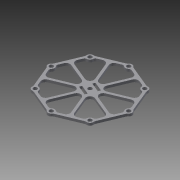
# Autodesk Inventor part: RPiConnector
Saved by Autodesk Inventor 2014 SP1 (Build 180222100, 222)
## iProperties
Created: 2014-07-30
Part Number: RPiConnector
Material: Generic
Document SubType Name: Modeling
Designer: Ryan
Density: 1 g/cm^3
Appearance: Default
Author: Ryan
Autodesk Inventor part; units mm, degrees
ref_plane "YZ Plane" through (0, 0, 0) normal (1, 0, 0) x (0, 1, 0)
ref_plane "XZ Plane" through (0, 0, 0) normal (0, 1, 0) x (-1, 0, 0)
ref_plane "XY Plane" through (0, 0, 0) normal (0, 0, 1) x (1, 0, 0)
sketch "Middle Plate" plane through (0, 0, 0) normal (0, 0, 1) x (1, 0, 0)
  circle A0 centre (54.1802, 86) radius 1.6
  circle A1 centre (63.5, 108.5) radius 1.6
  circle A2 centre (86, 117.8198) radius 1.6
  circle A3 centre (108.5, 108.5) radius 1.6
  circle A4 centre (117.8198, 86) radius 1.6
  circle A5 centre (108.5, 63.5) radius 1.6
  circle A6 centre (63.5, 63.5) radius 1.6
  circle A7 centre (86, 54.1802) radius 1.6
  arc A8 (56.1767, 84.1823) -> (56.1767, 87.8177) centre (54.1802, 86) ccw
  arc A9 (55.8078, 89.9295) -> (56.1767, 87.8177) centre (57.6556, 89.1641) ccw
  arc A10 (56.1767, 84.1823) -> (55.8078, 82.0705) centre (57.6556, 82.8359) ccw
  arc A11 (63.6264, 105.803) -> (66.197, 108.3735) centre (63.5, 108.5) ccw
  arc A12 (63.6264, 105.803) -> (61.8724, 104.5705) centre (63.7201, 103.8052) ccw
  arc A13 (67.4295, 110.1276) -> (66.197, 108.3735) centre (68.1948, 108.2799) ccw
  arc A14 (84.1823, 115.8233) -> (87.8177, 115.8233) centre (86, 117.8198) ccw
  arc A15 (89.9295, 116.1922) -> (87.8177, 115.8233) centre (89.1641, 114.3444) ccw
  arc A16 (84.1823, 115.8233) -> (82.0705, 116.1922) centre (82.8359, 114.3444) ccw
  arc A17 (105.803, 108.3735) -> (108.3735, 105.803) centre (108.5, 108.5) ccw
  arc A18 (110.1276, 104.5705) -> (108.3735, 105.803) centre (108.2799, 103.8052) ccw
  arc A19 (105.803, 108.3735) -> (104.5705, 110.1276) centre (103.8052, 108.2799) ccw
  arc A20 (115.8233, 87.8177) -> (115.8233, 84.1823) centre (117.8198, 86) ccw
  arc A21 (116.1922, 82.0705) -> (115.8233, 84.1823) centre (114.3444, 82.8359) ccw
  arc A22 (115.8233, 87.8177) -> (116.1922, 89.9295) centre (114.3444, 89.1641) ccw
  arc A23 (66.197, 63.6265) -> (63.6264, 66.197) centre (63.5, 63.5) ccw
  arc A24 (61.8724, 67.4295) -> (63.6264, 66.197) centre (63.7201, 68.1948) ccw
  arc A25 (66.197, 63.6265) -> (67.4295, 61.8724) centre (68.1948, 63.7201) ccw
  arc A26 (87.8177, 56.1767) -> (84.1823, 56.1767) centre (86, 54.1802) ccw
  arc A27 (82.0705, 55.8078) -> (84.1823, 56.1767) centre (82.8359, 57.6556) ccw
  arc A28 (87.8177, 56.1767) -> (89.9295, 55.8078) centre (89.1641, 57.6556) ccw
  arc A29 (108.3735, 66.197) -> (105.803, 63.6265) centre (108.5, 63.5) ccw
  arc A30 (104.5705, 61.8724) -> (105.803, 63.6265) centre (103.8052, 63.7201) ccw
  arc A31 (108.3735, 66.197) -> (110.1276, 67.4295) centre (108.2799, 68.1948) ccw
  line L0 (55.8078, 82.0705) -> (61.8724, 67.4295)
  line L1 (67.4295, 61.8724) -> (82.0705, 55.8078)
  line L2 (89.9295, 55.8078) -> (104.5705, 61.8724)
  line L3 (110.1276, 67.4295) -> (116.1922, 82.0705)
  line L4 (116.1922, 89.9295) -> (110.1276, 104.5705)
  line L5 (104.5705, 110.1276) -> (89.9295, 116.1922)
  line L6 (82.0705, 116.1922) -> (67.4295, 110.1276)
  line L7 (61.8724, 104.5705) -> (55.8078, 89.9295)
  point P0 (86, 86)
sketch "Sketch1" plane through (0, 0, 0) normal (0, 1, 0) x (-1, 0, 0)
  arc A0 (66.197, 63.6265) -> (67.4295, 61.8724) centre (68.1948, 63.7201) ccw
  arc A1 (61.8724, 67.4295) -> (63.6264, 66.197) centre (63.7201, 68.1948) ccw
  line L0 (61.8724, 67.4295) -> (60.0246, 66.6641)
  line L1 (67.4295, 61.8724) -> (66.6641, 60.0246)
  arc A2 (82.0705, 55.8078) -> (84.1823, 56.1767) centre (82.8359, 57.6556) ccw
  arc A3 (87.8177, 56.1767) -> (89.9295, 55.8078) centre (89.1641, 57.6556) ccw
  arc A4 (104.5705, 61.8724) -> (105.803, 63.6265) centre (103.8052, 63.7201) ccw
  arc A5 (108.3735, 66.197) -> (110.1276, 67.4295) centre (108.2799, 68.1948) ccw
  line L2 (67.4295, 61.8724) -> (82.0705, 55.8078)
  line L3 (82.0705, 55.8078) -> (81.3052, 53.9601)
  line L4 (81.3052, 53.9601) -> (66.6641, 60.0246)
  line L5 (89.9295, 55.8078) -> (104.5705, 61.8724)
  arc A6 (56.1767, 84.1823) -> (55.8078, 82.0705) centre (57.6556, 82.8359) ccw
  arc A7 (55.8078, 89.9295) -> (56.1767, 87.8177) centre (57.6556, 89.1641) ccw
  arc A8 (63.6264, 105.803) -> (61.8724, 104.5705) centre (63.7201, 103.8052) ccw
  arc A9 (67.4295, 110.1276) -> (66.197, 108.3735) centre (68.1948, 108.2799) ccw
  arc A10 (84.1823, 115.8233) -> (82.0705, 116.1922) centre (82.8359, 114.3444) ccw
  arc A11 (89.9295, 116.1922) -> (87.8177, 115.8233) centre (89.1641, 114.3444) ccw
  arc A12 (105.803, 108.3735) -> (104.5705, 110.1276) centre (103.8052, 108.2799) ccw
  arc A13 (110.1276, 104.5705) -> (108.3735, 105.803) centre (108.2799, 103.8052) ccw
  arc A14 (115.8233, 87.8177) -> (116.1922, 89.9295) centre (114.3444, 89.1641) ccw
  arc A15 (116.1922, 82.0705) -> (115.8233, 84.1823) centre (114.3444, 82.8359) ccw
  line L6 (110.1276, 67.4295) -> (116.1922, 82.0705)
  line L7 (116.1922, 89.9295) -> (110.1276, 104.5705)
  line L8 (104.5705, 110.1276) -> (89.9295, 116.1922)
  line L9 (82.0705, 116.1922) -> (67.4295, 110.1276)
  line L10 (61.8724, 104.5705) -> (55.8078, 89.9295)
  line L11 (55.8078, 82.0705) -> (61.8724, 67.4295)
  line L12 (55.8078, 82.0705) -> (53.9601, 81.3052)
  line L13 (55.8078, 89.9295) -> (53.9601, 90.6948)
  line L14 (61.8724, 104.5705) -> (60.0246, 105.3359)
  line L15 (60.0246, 105.3359) -> (53.9601, 90.6948)
  line L16 (60.0246, 66.6641) -> (53.9601, 81.3052)
  line L17 (89.9295, 55.8078) -> (90.6948, 53.9601)
  line L18 (104.5705, 61.8724) -> (105.3359, 60.0246)
  line L19 (90.6948, 53.9601) -> (105.3359, 60.0246)
  line L20 (110.1276, 67.4295) -> (111.9754, 66.6641)
  line L21 (116.1922, 82.0705) -> (118.0399, 81.3052)
  line L22 (118.0399, 81.3052) -> (111.9754, 66.6641)
  line L23 (116.1922, 89.9295) -> (118.0399, 90.6948)
  line L24 (110.1276, 104.5705) -> (111.9754, 105.3359)
  line L25 (111.9754, 105.3359) -> (118.0399, 90.6948)
  line L26 (104.5705, 110.1276) -> (105.3359, 111.9754)
  line L27 (89.9295, 116.1922) -> (90.6948, 118.0399)
  line L28 (90.6948, 118.0399) -> (105.3359, 111.9754)
  line L29 (82.0705, 116.1922) -> (81.3052, 118.0399)
  line L30 (67.4295, 110.1276) -> (66.6641, 111.9754)
  line L31 (66.6641, 111.9754) -> (81.3052, 118.0399)
  line L32 (60.0246, 105.3359) -> (60.9581, 107.5896)
  line L33 (66.6641, 111.9754) -> (64.4104, 111.0419)
  line L34 (90.6948, 118.0399) -> (88.4411, 118.9734)
  line L35 (81.3052, 118.0399) -> (83.5589, 118.9734)
  line L36 (105.3359, 111.9754) -> (107.5896, 111.0419)
  line L37 (111.9754, 105.3359) -> (111.0419, 107.5896)
  line L38 (118.0399, 90.6948) -> (118.9734, 88.4411)
  line L39 (118.0399, 81.3052) -> (118.9734, 83.5589)
  line L40 (111.9754, 66.6641) -> (111.0419, 64.4104)
  line L41 (105.3359, 60.0246) -> (107.5896, 60.9581)
  line L42 (81.3052, 53.9601) -> (83.5589, 53.0266)
  line L43 (90.6948, 53.9601) -> (88.4411, 53.0266)
  line L44 (66.6641, 60.0246) -> (64.4104, 60.9581)
  line L45 (60.0246, 66.6641) -> (60.9581, 64.4104)
  line L46 (53.9601, 81.3052) -> (53.0266, 83.5589)
  line L47 (53.9601, 90.6948) -> (53.0266, 88.4411)
  circle A16 centre (54.1802, 86) radius 1.6
  circle A17 centre (63.5, 108.5) radius 1.6
  circle A18 centre (86, 117.8198) radius 1.6
  circle A19 centre (108.5, 108.5) radius 1.6
  circle A20 centre (117.8198, 86) radius 1.6
  circle A21 centre (108.5, 63.5) radius 1.6
  circle A22 centre (86, 54.1802) radius 1.6
  arc A23 (56.1767, 84.1823) -> (55.8078, 82.0705) centre (57.6556, 82.8359) ccw
  arc A24 (55.8078, 89.9295) -> (56.1767, 87.8177) centre (57.6556, 89.1641) ccw
  arc A25 (63.6264, 105.803) -> (61.8724, 104.5705) centre (63.7201, 103.8052) ccw
  arc A26 (67.4295, 110.1276) -> (66.197, 108.3735) centre (68.1948, 108.2799) ccw
  arc A27 (84.1823, 115.8233) -> (82.0705, 116.1922) centre (82.8359, 114.3444) ccw
  arc A28 (89.9295, 116.1922) -> (87.8177, 115.8233) centre (89.1641, 114.3444) ccw
  arc A29 (105.803, 108.3735) -> (104.5705, 110.1276) centre (103.8052, 108.2799) ccw
  arc A30 (110.1276, 104.5705) -> (108.3735, 105.803) centre (108.2799, 103.8052) ccw
  arc A31 (115.8233, 87.8177) -> (116.1922, 89.9295) centre (114.3444, 89.1641) ccw
  arc A32 (116.1922, 82.0705) -> (115.8233, 84.1823) centre (114.3444, 82.8359) ccw
  arc A33 (108.3735, 66.197) -> (110.1276, 67.4295) centre (108.2799, 68.1948) ccw
  arc A34 (104.5705, 61.8724) -> (105.803, 63.6265) centre (103.8052, 63.7201) ccw
  arc A35 (87.8177, 56.1767) -> (89.9295, 55.8078) centre (89.1641, 57.6556) ccw
  arc A36 (82.0705, 55.8078) -> (84.1823, 56.1767) centre (82.8359, 57.6556) ccw
  arc A37 (66.1912, 63.7184) -> (67.4295, 61.8724) centre (68.2018, 63.7288) ccw
  arc A38 (61.8724, 67.4295) -> (63.6264, 66.197) centre (63.7201, 68.1948) ccw
  arc A39 (87.8177, 56.1767) -> (84.1823, 56.1767) centre (86, 54.1802) ccw
  arc A40 (83.5589, 53.0266) -> (88.4411, 53.0266) centre (86, 54.1802) ccw
  arc A41 (66.1912, 63.7184) -> (63.6264, 66.197) centre (63.5, 63.5) ccw
  arc A42 (60.9581, 64.4104) -> (64.4104, 60.9581) centre (63.5, 63.5) ccw
  arc A43 (108.3735, 66.197) -> (105.803, 63.6265) centre (108.5, 63.5) ccw
  arc A44 (107.5896, 60.9581) -> (111.0419, 64.4104) centre (108.5, 63.5) ccw
  arc A45 (115.8233, 87.8177) -> (115.8233, 84.1823) centre (117.8198, 86) ccw
  arc A46 (118.9734, 83.5589) -> (118.9734, 88.4411) centre (117.8198, 86) ccw
  arc A47 (105.803, 108.3735) -> (108.3735, 105.803) centre (108.5, 108.5) ccw
  arc A48 (111.0419, 107.5896) -> (107.5896, 111.0419) centre (108.5, 108.5) ccw
  arc A49 (84.1823, 115.8233) -> (87.8177, 115.8233) centre (86, 117.8198) ccw
  arc A50 (88.4411, 118.9734) -> (83.5589, 118.9734) centre (86, 117.8198) ccw
  arc A51 (63.6264, 105.803) -> (66.197, 108.3735) centre (63.5, 108.5) ccw
  arc A52 (64.4104, 111.0419) -> (60.9581, 107.5896) centre (63.5, 108.5) ccw
  arc A53 (53.0266, 88.4411) -> (53.0266, 83.5589) centre (54.1802, 86) ccw
  arc A54 (56.1767, 84.1823) -> (56.1767, 87.8177) centre (54.1802, 86) ccw
  circle A55 centre (63.5, 63.5) radius 1.6
  circle A56 centre (54.1802, 86) radius 1.6
  circle A57 centre (63.5, 108.5) radius 1.6
  circle A58 centre (86, 117.8198) radius 1.6
  circle A59 centre (108.5, 108.5) radius 1.6
  circle A60 centre (117.8198, 86) radius 1.6
  circle A61 centre (108.5, 63.5) radius 1.6
  circle A62 centre (63.5, 63.5) radius 1.6
  circle A63 centre (86, 54.1802) radius 1.6
  arc A64 (56.1767, 84.1823) -> (56.1767, 87.8177) centre (54.1802, 86) ccw
  arc A65 (55.8078, 89.9295) -> (56.1767, 87.8177) centre (57.6556, 89.1641) ccw
  arc A66 (56.1767, 84.1823) -> (55.8078, 82.0705) centre (57.6556, 82.8359) ccw
  arc A67 (63.6264, 105.803) -> (66.197, 108.3735) centre (63.5, 108.5) ccw
  arc A68 (63.6264, 105.803) -> (61.8724, 104.5705) centre (63.7201, 103.8052) ccw
  arc A69 (67.4295, 110.1276) -> (66.197, 108.3735) centre (68.1948, 108.2799) ccw
  arc A70 (84.1823, 115.8233) -> (87.8177, 115.8233) centre (86, 117.8198) ccw
  arc A71 (89.9295, 116.1922) -> (87.8177, 115.8233) centre (89.1641, 114.3444) ccw
  arc A72 (84.1823, 115.8233) -> (82.0705, 116.1922) centre (82.8359, 114.3444) ccw
  arc A73 (105.803, 108.3735) -> (108.3735, 105.803) centre (108.5, 108.5) ccw
  arc A74 (110.1276, 104.5705) -> (108.3735, 105.803) centre (108.2799, 103.8052) ccw
  arc A75 (105.803, 108.3735) -> (104.5705, 110.1276) centre (103.8052, 108.2799) ccw
  arc A76 (115.8233, 87.8177) -> (115.8233, 84.1823) centre (117.8198, 86) ccw
  arc A77 (116.1922, 82.0705) -> (115.8233, 84.1823) centre (114.3444, 82.8359) ccw
  arc A78 (115.8233, 87.8177) -> (116.1922, 89.9295) centre (114.3444, 89.1641) ccw
  arc A79 (66.197, 63.6265) -> (63.6264, 66.197) centre (63.5, 63.5) ccw
  arc A80 (61.8724, 67.4295) -> (63.6264, 66.197) centre (63.7201, 68.1948) ccw
  arc A81 (66.197, 63.6265) -> (67.4295, 61.8724) centre (68.1948, 63.7201) ccw
  arc A82 (87.8177, 56.1767) -> (84.1823, 56.1767) centre (86, 54.1802) ccw
  arc A83 (82.0705, 55.8078) -> (84.1823, 56.1767) centre (82.8359, 57.6556) ccw
  arc A84 (87.8177, 56.1767) -> (89.9295, 55.8078) centre (89.1641, 57.6556) ccw
  arc A85 (108.3735, 66.197) -> (105.803, 63.6265) centre (108.5, 63.5) ccw
  arc A86 (104.5705, 61.8724) -> (105.803, 63.6265) centre (103.8052, 63.7201) ccw
  arc A87 (108.3735, 66.197) -> (110.1276, 67.4295) centre (108.2799, 68.1948) ccw
  line L48 (55.8078, 82.0705) -> (61.8724, 67.4295)
  line L49 (67.4295, 61.8724) -> (82.0705, 55.8078)
  line L50 (89.9295, 55.8078) -> (104.5705, 61.8724)
  line L51 (110.1276, 67.4295) -> (116.1922, 82.0705)
  line L52 (116.1922, 89.9295) -> (110.1276, 104.5705)
  line L53 (104.5705, 110.1276) -> (89.9295, 116.1922)
  line L54 (82.0705, 116.1922) -> (67.4295, 110.1276)
  line L55 (61.8724, 104.5705) -> (55.8078, 89.9295)
  point P0 (0, 0)
  dimension "d1" = 2
  dimension "d2" = 2
  dimension "d3" = 2
  dimension "d4" = 2
  dimension "d5" = 2
  dimension "d6" = 2
  dimension "d7" = 2
  dimension "d8" = 2
  dimension "d9" = 2
  dimension "d10" = 2
  dimension "d11" = 2
  dimension "d12" = 2
  dimension "d13" = 2
  dimension "d14" = 2
  dimension "d15" = 2
  dimension "d16" = 2
  dimension "d19" = 90
  constraints: 96 end point, 96 point on circle, 56 centre point, 16 coincident, 15 perpendicular, 15 tangent, 9 parallel, 7 collinear, 6 concentric, 65 other
  measures "d1" distance of L0.start L0.end
  measures "d2" distance of L1.start L1.end
  measures "d3" distance of L2.end L3.end
  measures "d4" distance of L11.start L12.end
  measures "d5" distance of L10.end L13.end
  measures "d6" distance of L10.start L14.end
  measures "d7" distance of L5.start L17.end
  measures "d8" distance of L5.end L18.end
  measures "d9" distance of L6.start L20.end
  measures "d10" distance of L6.end L21.end
  measures "d11" distance of L7.start L23.end
  measures "d12" distance of L7.end L24.end
  measures "d13" distance of L8.start L26.end
  measures "d14" distance of L8.end L27.end
  measures "d15" distance of L9.start L29.end
  measures "d16" distance of L9.end L30.end
  measures "d19" angle of L1 L44
extrude "Extrusion1" add sketch "Sketch1" along normal blind 2 contours L1 L44 A42 L45 L0 A1 A41 A37 | L2 L3 L4 L1 | A2 A39 A3 L17 L43 A40 L42 L3 | L0 L16 L12 L11 | L12 L46 A53 L47 L13 A7 A54 A6 | L5 L18 L19 L17 | A4 A43 A5 L20 L40 A44 L41 L18 | L13 L15 L14 L10 | L14 L32 A52 L33 L30 A9 A51 A8 | L6 L21 L22 L20 | A15 A45 A14 L23 L38 A46 L39 L21 | L30 L31 L29 L9 | L29 L35 A50 L34 L27 A11 A49 A10 | L7 L24 L25 L23 | A13 A47 A12 L26 L36 A48 L37 L24 | L27 L28 L26 L8
fillet "Fillet1" radius 3.175 16 edges at (-53.0266, 1, 88.4411) (-53.0266, 1, 83.5589) (-60.9581, 1, 107.5896) (-64.4104, 1, 111.0419) (-83.5589, 1, 118.9734) (-88.4411, 1, 118.9734) (-107.5896, 1, 111.0419) (-111.0419, 1, 107.5896) (-118.9734, 1, 88.4411) (-118.9734, 1, 83.5589) (-111.0419, 1, 64.4104) (-107.5896, 1, 60.9581) (-88.4411, 1, 53.0266) (-64.4104, 1, 60.9581) (-83.5589, 1, 53.0266) (-60.9581, 1, 64.4104)
sketch "Sketch2" plane through (0, 2, 0) normal (0, 1, 0) x (1, 0, 0)
  line L0 (-110.1276, -104.5705) -> (-116.1922, -89.9295) projected
  line L1 (-116.1922, -82.0705) -> (-110.1276, -67.4295) projected
  line L2 (-104.5705, -61.8724) -> (-89.9295, -55.8078) projected
  line L3 (-82.0705, -55.8078) -> (-67.4295, -61.8724) projected
  line L4 (-61.8724, -67.4295) -> (-55.8078, -82.0705) projected
  line L5 (-55.8078, -89.9295) -> (-61.8724, -104.5705) projected
  line L6 (-67.4295, -110.1276) -> (-82.0705, -116.1922) projected
  line L7 (-89.9295, -116.1922) -> (-104.5705, -110.1276) projected
  line L8 (-113.1599, -74.75) -> (-58.8401, -97.25)
  line L9 (-58.8401, -74.75) -> (-113.1599, -97.25)
  line L10 (-97.25, -58.8401) -> (-74.75, -113.1599)
  line L11 (-74.75, -58.8401) -> (-97.25, -113.1599)
  line L12 (-97.25, -113.1599) -> (-96.3261, -113.5426)
  line L13 (-96.3261, -113.5426) -> (-73.8261, -59.2228)
  line L14 (-74.75, -58.8401) -> (-73.8261, -59.2228)
  line L15 (-74.75, -58.8401) -> (-75.6739, -58.4574)
  line L16 (-75.6739, -58.4574) -> (-98.1739, -112.7772)
  line L17 (-97.25, -113.1599) -> (-98.1739, -112.7772)
  line L18 (-74.75, -113.1599) -> (-73.8261, -112.7772)
  line L19 (-73.8261, -112.7772) -> (-96.3261, -58.4574)
  line L20 (-96.3261, -58.4574) -> (-98.1739, -59.2228)
  line L21 (-98.1739, -59.2228) -> (-75.6739, -113.5426)
  line L22 (-74.75, -113.1599) -> (-75.6739, -113.5426)
  line L23 (-113.1599, -97.25) -> (-112.7772, -98.1739)
  line L24 (-112.7772, -98.1739) -> (-58.4574, -75.6739)
  line L25 (-58.4574, -75.6739) -> (-59.2228, -73.8261)
  line L26 (-59.2228, -73.8261) -> (-113.5426, -96.3261)
  line L27 (-113.1599, -97.25) -> (-113.5426, -96.3261)
  line L28 (-113.1599, -74.75) -> (-112.7772, -73.8261)
  line L29 (-112.7772, -73.8261) -> (-58.4574, -96.3261)
  line L30 (-58.4574, -96.3261) -> (-59.2228, -98.1739)
  line L31 (-59.2228, -98.1739) -> (-113.5426, -75.6739)
  line L32 (-113.1599, -74.75) -> (-113.5426, -75.6739)
  point P0 (0, 0)
  dimension "d23" = 1
  dimension "d24" = 1
  dimension "d25" = 1
  dimension "d26" = 2
  dimension "d27" = 1
  dimension "d28" = 2
  dimension "d29" = 1
  dimension "d30" = 2
  constraints: 50 end point, 16 point on line, 9 midpoint, 9 perpendicular, 3 collinear
  measures "d23" distance of L11.end L12.end
  measures "d24" distance of L11.start L15.end
  measures "d25" distance of L10.end L18.end
  measures "d26" distance of L19.end L20.end
  measures "d27" distance of L9.end L23.end
  measures "d28" distance of L24.end L25.end
  measures "d29" distance of L8.start L28.end
  measures "d30" distance of L29.end L30.end
extrude "Extrusion2" add sketch "Sketch2" against normal blind 2
fillet "Fillet2" radius 3.175 24 edges at (-86, 1, 88.6131) (-84.1522, 1, 87.8478) (-83.3869, 1, 86) (-84.1522, 1, 84.1522) (-86, 1, 83.3869) (-87.8478, 1, 84.1522) (-88.6131, 1, 86) (-75.6739, 1, 113.5426) (-73.8261, 1, 112.7772) (-98.1739, 1, 112.7772) (-96.3261, 1, 113.5426) (-113.5426, 1, 96.3261) (-112.7772, 1, 98.1739) (-112.7772, 1, 73.8261) (-113.5426, 1, 75.6739) (-96.3261, 1, 58.4574) (-98.1739, 1, 59.2228) (-73.8261, 1, 59.2228) (-87.8478, 1, 87.8478) (-75.6739, 1, 58.4574) (-58.4574, 1, 75.6739) (-59.2228, 1, 98.1739) (-58.4574, 1, 96.3261) (-59.2228, 1, 73.8261)
sketch "Sketch3" plane through (0, 2, 0) normal (0, 1, 0) x (1, 0, 0)
  arc A0 (-76.3052, -83.0667) -> (-76.3052, -88.9333) centre (-75.0902, -86) ccw projected
  arc A1 (-90.7811, -94.9294) -> (-94.9294, -90.7811) centre (-93.7144, -93.7144) ccw projected
  arc A2 (-94.9294, -81.2189) -> (-90.7811, -77.0706) centre (-93.7144, -78.2856) ccw projected
  arc A3 (-77.0706, -90.7811) -> (-81.2189, -94.9294) centre (-78.2856, -93.7144) ccw projected
  arc A4 (-83.0667, -95.6948) -> (-88.9333, -95.6948) centre (-86, -96.9098) ccw projected
  arc A5 (-95.6948, -88.9333) -> (-95.6948, -83.0667) centre (-96.9098, -86) ccw projected
  arc A6 (-81.2189, -77.0706) -> (-77.0706, -81.2189) centre (-78.2856, -78.2856) ccw projected
  arc A7 (-88.9333, -76.3052) -> (-83.0667, -76.3052) centre (-86, -75.0902) ccw projected
  line L0 (-82.0705, -55.8078) -> (-78.6072, -57.2424) projected
  circle A8 centre (-86, -86) radius 1.6002
  line L1 (-93.7144, -93.7144) -> (-86, -75.0902)
  line L2 (-78.2856, -78.2856) -> (-86, -96.9098)
  line L3 (-78.2856, -93.7144) -> (-96.9098, -86)
  line L4 (-93.7144, -78.2856) -> (-75.0902, -86)
  line L5 (-91.4549, -88.2595) -> (-91.8296, -89.1641)
  line L6 (-91.8296, -89.1641) -> (-84.1152, -92.3595)
  line L7 (-84.1152, -92.3595) -> (-83.357, -90.5291)
  line L8 (-83.357, -90.5291) -> (-91.0714, -87.3337)
  line L9 (-91.8296, -89.1641) -> (-91.0714, -87.3337)
  line L10 (-88.2595, -80.5451) -> (-87.8804, -79.6299)
  line L11 (-87.8804, -79.6299) -> (-80.166, -82.8253)
  line L12 (-80.166, -82.8253) -> (-80.9242, -84.6557)
  line L13 (-80.9242, -84.6557) -> (-88.6386, -81.4603)
  line L14 (-87.8804, -79.6299) -> (-88.6386, -81.4603)
  point P0 (0, 0)
  dimension "d34" = 3.2004
  dimension "d37" = 1.9812
  dimension "d38" = 0.9906
  dimension "d39" = 1.9812
  constraints: 28 end point, 12 point on line, 6 perpendicular, 2 collinear, 2 parallel, 1 centre point
  measures "d34" diameter of A8
  measures "d37" distance of L6.end L7.end
  measures "d38" distance of L10.start L10.end
  measures "d39" distance of L11.end L12.end
extrude "Extrusion3" cut sketch "Sketch3" against normal blind 2 contours A8 | L1 L3 L2 L6 | L1 L8 L2 L3 | L1 L4 L2 L13 | L1 L11 L2 L4
body "Solid1"
